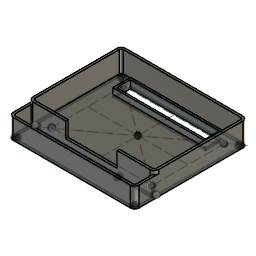
Amoled 2.41 v1 (Autodesk Fusion 360 design; units mm, degrees)
part number: 2026-08-13-11-23-48-228
Autodesk Fusion 360 part; units mm, degrees
sketch "Esquisse1" plane through (0, 0, 0) normal (0, 0, 1) x (1, 0, 0)
  line L0 (0, 0) -> (51, 0) construction
  line L1 (51, 0) -> (51, 36.5) construction
  line L2 (51, 36.5) -> (0, 36.5) construction
  line L3 (0, 36.5) -> (0, 0) construction
  circle A0 centre (0, 36.5) radius 1.2
  circle A1 centre (51, 36.5) radius 1.2
  circle A2 centre (0, 0) radius 1.2
  circle A3 centre (51, 0) radius 1.2
  line L4 (0, 18.25) -> (51, 18.25) construction
  line L5 (25.5, 36.5) -> (25.5, 0) construction
  line L6 (55.28, 41.85) -> (-4.28, 41.85)
  line L7 (-6.5, 39.63) -> (-6.5, -3.13)
  line L8 (-4.28, -5.35) -> (55.28, -5.35)
  line L9 (57.5, -3.13) -> (57.5, 39.63)
  line L10 (57.5, 41.85) -> (-6.5, -5.35) construction
  line L11 (-6.5, 41.85) -> (57.5, -5.35) construction
  line L12 (50.325, 36.86) -> (0.675, -0.36) construction
  line L13 (0.675, 36.86) -> (50.325, -0.36) construction
  line L14 (-5.3, 39.65) -> (-5.3, -3.15)
  line L15 (-4.3, -4.15) -> (55.3, -4.15)
  line L16 (56.3, -3.15) -> (56.3, 39.65)
  line L17 (55.3, 40.65) -> (-4.3, 40.65)
  arc A4 (-4.3, 40.65) -> (-5.3, 39.65) centre (-4.3, 39.65) ccw
  arc A5 (56.3, 39.65) -> (55.3, 40.65) centre (55.3, 39.65) ccw
  arc A6 (55.3, -4.15) -> (56.3, -3.15) centre (55.3, -3.15) ccw
  arc A7 (-5.3, -3.15) -> (-4.3, -4.15) centre (-4.3, -3.15) ccw
  arc A8 (57.5, 39.63) -> (55.28, 41.85) centre (55.28, 39.63) ccw
  arc A9 (-4.28, 41.85) -> (-6.5, 39.63) centre (-4.28, 39.63) ccw
  arc A10 (-6.5, -3.13) -> (-4.28, -5.35) centre (-4.28, -3.13) ccw
  arc A11 (55.28, -5.35) -> (57.5, -3.13) centre (55.28, -3.13) ccw
  line L18 (3, 37.05) -> (48, 37.05)
  line L19 (48, 37.05) -> (48, 30.05)
  line L20 (48, 30.05) -> (3, 30.05)
  line L21 (3, 30.05) -> (3, 37.05)
  line L22 (2, 38.05) -> (49, 38.05)
  line L23 (49, 38.05) -> (49, 29.05)
  line L24 (49, 29.05) -> (2, 29.05)
  line L25 (2, 29.05) -> (2, 38.05)
  line L26 (12.5, -4.15) -> (12.5, -5.35)
  line L27 (38.5, -4.15) -> (38.5, -5.35)
  line L28 (57.5, -3.13) -> (57.5, -13.13)
  line L29 (55.28, -15.35) -> (-4.28, -15.35)
  line L30 (-6.5, -13.13) -> (-6.5, -3.13)
  line L31 (56.3, -3.13) -> (56.3, -13.15)
  line L32 (55.3, -14.15) -> (-4.3, -14.15)
  line L33 (-5.3, -13.15) -> (-5.3, -3.13)
  arc A12 (-5.3, -13.15) -> (-4.3, -14.15) centre (-4.3, -13.15) ccw
  arc A13 (55.3, -14.15) -> (56.3, -13.15) centre (55.3, -13.15) ccw
  arc A14 (55.28, -15.35) -> (57.5, -13.13) centre (55.28, -13.13) ccw
  arc A15 (-6.5, -13.13) -> (-4.28, -15.35) centre (-4.28, -13.13) ccw
  point P0 (25.5, 18.25)
  point P1 (25.5, 18.25)
  dimension "d1" = 51
  dimension "d2" = 36.5
  dimension "d3" = 2.4
  dimension "d4" = 2.4
  dimension "d5" = 2.4
  dimension "d6" = 2.4
  dimension "d7" = 64
  dimension "d8" = 47.2
  dimension "d9" = 49.65
  dimension "d10" = 37.22
  dimension "d16" = 1
  dimension "d17" = 2.22
  dimension "d21" = 9.5
  dimension "d22" = 9.5
  dimension "d23" = 4.8
  dimension "d24" = 11.8
  dimension "d25" = -1
  dimension "d28" = 13
  dimension "d29" = 10
  dimension "d31" = 1
  dimension "d32" = 2.22
  constraint horizontal L0
  constraint vertical L1
  constraint horizontal L2
  constraint vertical L3
  constraint coincident L0.start L3.end
  constraint coincident L2.end L3.start
  constraint coincident L1.end L2.start
  constraint coincident L0.end L1.start
  constraint midpoint L3 L4.start
  constraint midpoint L1 L4.end
  constraint midpoint L2 L5.start
  constraint midpoint L0 L5.end
  constraint horizontal L6
  constraint perpendicular L6 L7
  constraint parallel L6 L8
  constraint parallel L7 L9
  constraint coincident L10 P1
  constraint coincident L11 P1
  constraint midpoint L5 P1
  constraint coincident L12 P1
  constraint coincident L13 P1
  constraint coincident P1 P0
  constraint tangent L14 A4
  constraint tangent L17 A4
  constraint tangent L16 A5
  constraint tangent L17 A5
  constraint equal A4 A5
  constraint tangent L15 A6
  constraint tangent L16 A6
  constraint equal A4 A6
  constraint tangent L14 A7
  constraint tangent L15 A7
  constraint equal A4 A7
  constraint coincident L10.start L6
  constraint coincident L10.start L9
  constraint tangent L6 A8
  constraint tangent L9 A8
  constraint coincident L11.start L7
  constraint coincident L11.start L6
  constraint tangent L7 A9
  constraint tangent L6 A9
  constraint equal A8 A9
  constraint coincident L10.end L7
  constraint coincident L10.end L8
  constraint tangent L7 A10
  constraint tangent L8 A10
  constraint equal A8 A10
  constraint coincident L11.end L8
  constraint coincident L11.end L9
  constraint tangent L8 A11
  constraint tangent L9 A11
  constraint equal A8 A11
  constraint horizontal L18
  constraint vertical L19
  constraint horizontal L20
  constraint vertical L21
  constraint coincident L15 L26.start
  constraint coincident L8 L26.end
  constraint perpendicular L8 L26
  constraint symmetric L5 L26.start L27.start
  constraint symmetric L5 L26.end L27.end
  constraint tangent A11 L28
  constraint tangent A10 L30
  constraint horizontal L29
  constraint tangent L32 A12
  constraint tangent L33 A12
  constraint tangent L31 A13
  constraint tangent L32 A13
  constraint equal A12 A13
  constraint tangent L28 A14
  constraint tangent L29 A14
  constraint tangent L29 A15
  constraint tangent L30 A15
  constraint equal A14 A15
  measures "d1" distance of L0.start L0.end
  measures "d2" distance of L0.start L2.end
  measures "d3" diameter of A0
  measures "d4" diameter of A1
  measures "d5" diameter of A2
  measures "d6" diameter of A3
  measures "d7" distance of L10.end L11.end
  measures "d8" distance of L11.start L10.end
  measures "d9" distance of L12.end L13.end
  measures "d10" distance of L13.start L12.end
  measures "d16" radius of A4
  measures "d17" radius of A8
  measures "d21" distance of L7 L21
  measures "d22" distance of L9 L19
  measures "d23" distance of L6 L18
  measures "d24" distance of L6 L20
  measures "d28" distance of L5 L26
  measures "d29" distance of L8 L29
  measures "d31" radius of A12
  measures "d32" radius of A14
extrude "Extrusion1" add sketch "Esquisse1" along normal blind 1 contours L8 A10 A11 L31 L32 L33 A12 A13 | L8 L15 A6 A11 L27 L31 | L8 L15 A7 A10 L26 L33 | L14 L15 L16 L17 A4 A5 A6 A7 L31 L33 | L8 L15 L26 L27 | L22 L23 L24 L25
extrude "Extrusion2" add sketch "Esquisse1" along normal blind 11.8 contours L6 L7 L9 L14 L16 L17 A4 A5 A8 A9 A10 A11 L31 L33 | L8 L15 A6 A11 L27 L31 | L8 L15 A7 A10 L26 L33
chamfer "Chanfrein1" distance 1 angle 45 4 edges at (-1.1188, 0.4339, 0) (49.8812, 0.4339, 0) (49.8812, 36.9339, 0) (-1.1188, 36.9339, 0)
extrude "Extrusion3" add sketch "Esquisse1" along normal blind 4 contours L8 L15 L26 L27 | L22 L23 L24 L25
extrude "Extrusion4" add sketch "Esquisse1" along normal blind 10 contours A10 A11 L28 L29 L30 L31 L32 L33 A12 A13 A14 A15
equation "d4 = d3"
equation "d5 = d3"
equation "d6 = d3"
